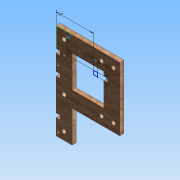
# Autodesk Inventor part: holdersupport
Saved by Autodesk Inventor 2015 (Build 190159000, 159)
## iProperties
Created: 2014-09-02
Part Number: holdersupport
Material: Wood (Birch)
Document SubType Name: Modeling
Designer: shohei
Density: 0.55 g/cm^3
Appearance: Birch - Natural Polished
Author: shohei
Autodesk Inventor part; units mm, degrees
note: some values were not read from the file. Chosen so that the rebuilt part matches the saved one: sketch regions of "Extrusion14".
ref_plane "YZ Plane" through (0, 0, 0) normal (1, 0, 0) x (0, 1, 0)
ref_plane "XZ Plane" through (0, 0, 0) normal (0, 1, 0) x (-1, 0, 0)
ref_plane "XY Plane" through (0, 0, 0) normal (0, 0, 1) x (1, 0, 0)
sketch "Sketch4" plane through (0, 0, 0) normal (0, 1, 0) x (-1, 0, 0)
  line L0 (0, 0) -> (20, 0)
  line L1 (20, 0) -> (20, 80)
  line L2 (20, 80) -> (0, 80)
  line L3 (0, 80) -> (0, 0)
  circle A0 centre (10, 10) radius 2.5
  circle A1 centre (10, 70) radius 2.5
  circle A2 centre (10, 70) radius 2.5
  line L4 (0, 0) -> (20, 0)
  line L5 (20, 0) -> (20, -40)
  line L6 (20, -40) -> (0, -40)
  line L7 (0, -40) -> (0, 0)
  circle A3 centre (10, -30) radius 2.5
  dimension "d0" = 80
  dimension "d3" = 20
  dimension "d4" = 5
  dimension "d5" = 10
  dimension "d6" = 10
  dimension "d7" = 5
  dimension "d8" = 10
  dimension "d9" = 10
  dimension "d12" = 5
  dimension "d13" = 60
  dimension "d16" = 40
  dimension "d17" = 5
  dimension "d18" = 10
  dimension "d19" = 10
  constraints: 16 end point, 4 centre point, 4 parallel, 2 horizontal, 2 perpendicular
  measures "d0" distance of L0.end L1.end
  measures "d3" distance of L1.end L2.end
  measures "d4" diameter of A0
  measures "d5" distance from line of L1 A0.centre
  measures "d6" distance from line of L0 A0.centre
  measures "d7" diameter of A1
  measures "d8" distance from line of L3 A1.centre
  measures "d9" distance from line of L2 A1.centre
  measures "d12" diameter of A2
  measures "d13" distance of A0.centre A2.centre
  measures "d16" distance of L4.end L5.end
  measures "d17" diameter of A3
  measures "d18" distance from line of L7 A3.centre
  measures "d19" distance from line of L6 A3.centre
extrude "Extrusion3" add sketch "Sketch4" along normal blind 5 contours L3 L2 L1 L0
sketch "Sketch5" plane through (0, 5, 0) normal (0, 1, 0) x (1, 0, 0)
  line L0 (60, -20) -> (-20, -20) projected
  line L1 (-20, -20) -> (-20, 0) projected
  line L2 (60, -20) -> (-20, -20) projected
  line L3 (60, 0) -> (60, -20) projected
  line L4 (-20, 0) -> (60, 0) projected
  circle A0 centre (-10, -70) radius 2.5 projected
  circle A1 centre (-10, -10) radius 2.5 projected
  line L5 (0, 0) -> (-20, 0) projected
  line L6 (-20, 0) -> (-20, -80) projected
  line L7 (-20, -80) -> (0, -80) projected
  line L8 (0, -80) -> (0, 0) projected
  line L9 (-20, 0) -> (0, 0)
  line L10 (0, 0) -> (0, 40)
  line L11 (0, 40) -> (-20, 40)
  line L12 (-20, 40) -> (-20, 0)
  circle A2 centre (-10, 30) radius 2.5
  circle A3 centre (50, -10) radius 2.5 projected
  circle A4 centre (-10, -10) radius 2.5 projected
  circle A5 centre (35, -10) radius 2.5 projected
  dimension "d20" = 40
  dimension "d21" = 5
  dimension "d22" = 10
  dimension "d23" = 10
  constraints: 8 end point, 2 parallel, 1 centre point, 1 horizontal, 1 perpendicular
  measures "d20" distance of L11.end L5.end
  measures "d21" diameter of A2
  measures "d22" distance from line of L10 A2.centre
  measures "d23" distance from line of L11 A2.centre
extrude "Extrusion4" add sketch "Sketch5" against normal blind 5 contours L4 L12 L11 L10
sketch "Sketch6" plane through (0, 5, 0) normal (0, 1, 0) x (1, 0, 0)
  line L0 (-20, 15) -> (-15, 15)
  line L1 (-15, 15) -> (-15, 20)
  line L2 (-15, 20) -> (-20, 20)
  line L3 (-20, 20) -> (-20, 15)
  line L4 (-20, 15) -> (-15, 20) construction
  line L5 (-15, 15) -> (-20, 20) construction
  line L6 (0, 40) -> (-20, 40) projected
  line L7 (-20, 40) -> (-20, -80) projected
  line L8 (-20, -25) -> (-15, -25)
  line L9 (-15, -25) -> (-15, -30)
  line L10 (-15, -30) -> (-20, -30)
  line L11 (-20, -30) -> (-20, -25)
  line L12 (-20, -25) -> (-15, -30) construction
  line L13 (-15, -25) -> (-20, -30) construction
  point P0 (0, 0)
  point P1 (-17.5, 17.5)
  point P2 (-17.5, -27.5)
  dimension "d26" = 5
  dimension "d27" = 5
  dimension "d28" = 20
  dimension "d29" = 5
  dimension "d30" = 5
  dimension "d31" = 40
  constraints: 24 end point, 4 midpoint, 4 parallel, 2 collinear, 2 horizontal, 2 perpendicular
  measures "d26" distance of L2.end L1.end
  measures "d27" distance of L1.end L0.end
  measures "d28" distance between parallel lines of L6 L2
  measures "d29" distance of L9.end L10.end
  measures "d30" distance of L8.end L9.end
  measures "d31" distance between parallel lines of L0 L8
extrude "Extrusion5" cut sketch "Sketch6" against normal through all
sketch "Sketch7" plane through (0, 5, 0) normal (0, 1, 0) x (1, 0, 0)
  circle A0 centre (-10, -52.5) radius 1
  line L0 (-20, -30) -> (-20, -80) projected
  line L1 (0, 40) -> (-20, 40) projected
  point P0 (0, 0)
  dimension "d34" = 2
  dimension "d35" = 10
  dimension "d36" = 92.5
  constraints: 1 centre point
  measures "d34" diameter of A0
  measures "d35" distance from line of L0 A0.centre
  measures "d36" distance from line of L1 A0.centre
extrude "Extrusion6" cut sketch "Sketch7" against normal through all
sketch "Sketch8" plane through (0, 0, 0) normal (0, -1, 0) x (1, 0, 0)
  circle A0 centre (-17.5, -35) radius 1
  line L0 (-20, -20) -> (-20, -40) projected
  line L1 (-20, -40) -> (0, -40) projected
  point P0 (0, 0)
  dimension "d39" = 2
  dimension "d40" = 2.5
  dimension "d41" = 5
  constraints: 1 centre point
  measures "d39" diameter of A0
  measures "d40" distance from line of L0 A0.centre
  measures "d41" distance from line of L1 A0.centre
extrude "Extrusion7" cut sketch "Sketch8" against normal through all
sketch "Sketch9" plane through (0, 0, 0) normal (0, -1, 0) x (1, 0, 0)
  circle A0 centre (-17.5, 38) radius 1
  line L0 (-20, 80) -> (-20, 30) projected
  line L1 (-20, 30) -> (-15, 30) projected
  point P0 (0, 0)
  dimension "d44" = 2
  dimension "d45" = 2.5
  dimension "d46" = 8
  constraints: 1 centre point
  measures "d44" diameter of A0
  measures "d45" distance from line of L0 A0.centre
  measures "d46" distance from line of L1 A0.centre
extrude "Extrusion8" cut sketch "Sketch9" against normal through all
sketch "Sketch10" plane through (0, 5, 0) normal (0, 1, 0) x (1, 0, 0)
  circle A0 centre (50, -70) radius 2.5 projected
  circle A1 centre (-10, -70) radius 2.5 projected
  circle A2 centre (35, -70) radius 2.5 projected
  line L0 (-20, -80) -> (-20, -60) projected
  line L1 (60, -80) -> (-20, -80) projected
  line L2 (60, -60) -> (60, -80) projected
  line L3 (-20, -60) -> (60, -60) projected
  circle A3 centre (50, -10) radius 2.5 projected
  circle A4 centre (35, -10) radius 2.5 projected
  circle A5 centre (50, -70) radius 2.5 projected
  circle A6 centre (35, -70) radius 2.5 projected
  line L4 (57, 0) -> (27, 0) projected
  line L5 (27, 0) -> (27, -80) projected
  line L6 (27, -80) -> (57, -80) projected
  line L7 (57, -80) -> (57, 0) projected
  circle A7 centre (50, -10) radius 2.5 projected
  circle A8 centre (-10, -10) radius 2.5 projected
  circle A9 centre (35, -10) radius 2.5 projected
  line L8 (-20, -20) -> (-20, 0) projected
  line L9 (60, -20) -> (-20, -20) projected
  line L10 (60, 0) -> (60, -20) projected
  line L11 (-20, 0) -> (60, 0) projected
  line L12 (-20, -80) -> (57, -80)
  line L13 (57, -80) -> (57, -60)
  line L14 (57, -60) -> (-20, -60)
  line L15 (-20, -60) -> (-20, -80)
  line L16 (57, 0) -> (27, 0)
  line L17 (27, 0) -> (27, -80)
  line L18 (27, -80) -> (57, -80)
  line L19 (57, -80) -> (57, 0)
  line L20 (-20, 0) -> (57, 0)
  line L21 (57, 0) -> (57, -20)
  line L22 (57, -20) -> (-20, -20)
  line L23 (-20, -20) -> (-20, 0)
  point P0 (0, 0)
  constraints: 24 end point, 6 parallel, 4 point on line, 3 horizontal, 3 perpendicular
extrude "Extrusion9" [suppressed]
sketch "Sketch11" plane through (0, 0, 0) normal (0, -1, 0) x (1, 0, 0)
  line L0 (-20, 55) -> (-15, 55)
  line L1 (-15, 55) -> (-15, 50)
  line L2 (-15, 50) -> (-20, 50)
  line L3 (-20, 50) -> (-20, 55)
  line L4 (-20, 80) -> (0, 80) projected
  line L5 (-20, 80) -> (-20, 30) projected
  point P0 (0, 0)
  point P1 (57, 80)
  dimension "d51" = 5
  dimension "d52" = 5
  dimension "d53" = 25
  constraints: 8 end point, 2 parallel, 1 collinear, 1 horizontal, 1 perpendicular
  measures "d51" distance of L1.end L2.end
  measures "d52" distance of L0.end L1.end
  measures "d53" distance between parallel lines of L4 L0
extrude "Extrusion10" cut sketch "Sketch11" against normal through all
sketch "Sketch12" plane through (0, 0, 0) normal (0, -1, 0) x (1, 0, 0)
  line L0 (27, 50) -> (32, 50)
  line L1 (32, 50) -> (32, 55)
  line L2 (32, 55) -> (27, 55)
  line L3 (27, 55) -> (27, 50)
  line L4 (-20, 80) -> (-20, 55) projected
  line L5 (-20, 80) -> (0, 80) projected
  point P0 (0, 0)
  point P1 (57, 80)
  dimension "d56" = 5
  dimension "d57" = 5
  dimension "d58" = 47
  dimension "d59" = 25
  constraints: 8 end point, 2 parallel, 1 horizontal, 1 perpendicular
  measures "d56" distance of L2.end L1.end
  measures "d57" distance of L1.end L0.end
  measures "d58" distance between parallel lines of L4 L3
  measures "d59" distance between parallel lines of L5 L2
sketch "Sketch15" plane through (0, 5, 0) normal (0, 1, 0) x (1, 0, 0)
  line L0 (-12.5, -55) -> (-12.5, -103) projected
  line L1 (-5.379, -59) -> (-8.621, -59) projected
  circle A0 centre (-10, -10) radius 2.5 projected
  circle A1 centre (-10, -70) radius 2.5 projected
  circle A2 centre (-10, 30) radius 2.5 projected
  line L2 (-20, -50) -> (-15, -50) projected
  line L3 (-15, -50) -> (-15, -55) projected
  line L4 (-15, -55) -> (-20, -55) projected
  line L5 (-20, -55) -> (-20, -80) projected
  line L6 (-20, -80) -> (0, -80) projected
  line L7 (0, -80) -> (0, 40) projected
  line L8 (0, 40) -> (-20, 40) projected
  line L9 (-20, 20) -> (-15, 20) projected
  line L10 (-15, 20) -> (-15, 15) projected
  line L11 (-15, 15) -> (-20, 15) projected
  line L12 (-20, 15) -> (-20, -25) projected
  line L13 (-20, -25) -> (-15, -25) projected
  line L14 (-15, -25) -> (-15, -30) projected
  line L15 (-15, -30) -> (-20, -30) projected
  line L16 (-20, -30) -> (-20, -50) projected
  circle A3 centre (-10, -52.5) radius 1 projected
  circle A4 centre (-17.5, 35) radius 1 projected
  circle A5 centre (-17.5, -38) radius 1 projected
  line L17 (-20, -80) -> (60, -80)
  line L18 (60, -80) -> (60, -60)
  line L19 (60, -60) -> (-20, -60)
  line L20 (-20, -60) -> (-20, -80)
  line L21 (60, -80) -> (40, -80)
  line L22 (40, -80) -> (40, 0)
  line L23 (40, 0) -> (60, 0)
  line L24 (60, 0) -> (60, -80)
  line L25 (-20, 0) -> (60, 0)
  line L26 (60, 0) -> (60, -20)
  line L27 (60, -20) -> (-20, -20)
  line L28 (-20, -20) -> (-20, 0)
  circle A6 centre (37, -70) radius 2.5
  circle A7 centre (52, -70) radius 2.5
  circle A8 centre (52, -10) radius 2.5
  circle A9 centre (37, -10) radius 2.5
  line L29 (-20, 40) -> (-20, 20) projected
  point P0 (0, 0)
  dimension "d69" = 20
  dimension "d70" = 80
  dimension "d71" = 20
  dimension "d72" = 80
  dimension "d73" = 5
  dimension "d74" = 5
  dimension "d75" = 8
  dimension "d76" = 23
  dimension "d77" = 5
  dimension "d78" = 5
  dimension "d79" = 8
  dimension "d80" = 23
  dimension "d81" = 10
  dimension "d82" = 10
  dimension "d90" = 20
  constraints: 24 end point, 6 parallel, 4 centre point, 3 horizontal, 3 perpendicular, 3 point on line
  measures "d69" distance between parallel lines of L19 L17
  measures "d70" distance between parallel lines of L18 L5
  measures "d71" distance between parallel lines of L25 L27
  measures "d72" distance between parallel lines of L26 L12
  measures "d73" diameter of A6
  measures "d74" diameter of A7
  measures "d75" distance from line of L24 A7.centre
  measures "d76" distance from line of L18 A6.centre
  measures "d77" diameter of A8
  measures "d78" diameter of A9
  measures "d79" distance from line of L24 A8.centre
  measures "d80" distance from line of L24 A9.centre
  measures "d81" distance from line of L23 A9.centre
  measures "d82" distance from line of L17 A6.centre
  measures "d90" distance between parallel lines of L24 L22
extrude "Extrusion14" add sketch "Sketch15" against normal blind 5 contours L19 L7 L6 L0 | L0 L6 L5 L19 | L19 L22 L17 L7 | L27 L12 L25 L7 | L7 L25 L22 L27 | L22 L27 L24 L19 | L19 L18 L17 L22 | L22 L23 L24 L27
sketch "Sketch16" plane through (0, 5, 0) normal (0, 1, 0) x (1, 0, 0)
  line L0 (45, -55) -> (40, -55)
  line L1 (40, -55) -> (40, -50)
  line L2 (40, -50) -> (45, -50)
  line L3 (45, -50) -> (45, -55)
  line L4 (40, -20) -> (40, -60) projected
  line L5 (-20, -80) -> (60, -80) projected
  point P0 (0, 0)
  dimension "d85" = 5
  dimension "d86" = 5
  dimension "d87" = 25
  constraints: 8 end point, 2 parallel, 1 collinear, 1 horizontal, 1 perpendicular
  measures "d85" distance of L1.end L2.end
  measures "d86" distance of L0.end L1.end
  measures "d87" distance between parallel lines of L5 L0
extrude "Extrusion15" cut sketch "Sketch16" against normal through all
equation "\"d37\" = d36"
body "Solid3"
